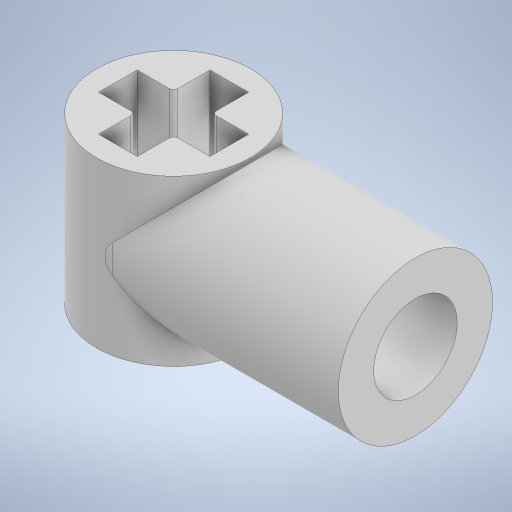
# Autodesk Inventor part: Part2
Saved by Autodesk Inventor 2024 (Build 280153000, 153)
## iProperties
Created: 2023-10-06
Part Number: Part2
Material: Generic
Document SubType Name: Modeling
Designer: kubad
Density: 1 g/cm^3
Appearance: Default
Author: kubad
## iProperties of the stored document Part2_3DPrint.ipt
Created: 2023-10-06
Part Number: Part2_3DPrint
Material: Generic
Document SubType Name: Modeling
Designer: kubad
Density: 1 g/cm^3
Appearance: Default
Author: kubad
Autodesk Inventor part; units mm, degrees
ref_plane "YZ Plane" through (0, 0, 0) normal (1, 0, 0) x (0, 1, 0)
ref_plane "XZ Plane" through (0, 0, 0) normal (0, 1, 0) x (-1, 0, 0)
ref_plane "XY Plane" through (0, 0, 0) normal (0, 0, 1) x (1, 0, 0)
sketch "Sketch1" plane through (0, 0, 0) normal (0, 1, 0) x (-1, 0, 0)
  point P0 (0, 0)
sketch "Sketch2" plane through (0, 0, 0) normal (0, 1, 0) x (-1, 0, 0)
  circle A0 centre (0, 0) radius 3.6
  dimension "d0" = 7.2
  constraints: 1 centre point, 1 coincident
  measures "d0" diameter of A0
extrude "Extrusion1" add sketch "Sketch2" along normal blind 7.7
sketch "Sketch3" plane through (0, 0, 0) normal (0, -1, 0) x (1, 0, 0)
  circle A0 centre (0, 0) radius 3.6 projected
  line L0 (0, 3.6) -> (3.6, 3.6)
  line L1 (3.6, 3.6) -> (3.6, -3.6)
  line L2 (3.6, -3.6) -> (0, -3.6)
  line L3 (0, -3.6) -> (0, 3.6)
  line L4 (3.6, 3.6) -> (11.4, 3.6)
  line L5 (11.4, 3.6) -> (11.4, -3.6)
  line L6 (11.4, -3.6) -> (3.6, -3.6)
  line L7 (3.6, -3.6) -> (3.6, 3.6)
  line L8 (11.4, 3.6) -> (11.3, 3.6)
  line L9 (11.3, 3.6) -> (11.3, -3.6)
  line L10 (11.3, -3.6) -> (11.4, -3.6)
  line L11 (11.4, -3.6) -> (11.4, 3.6)
  dimension "d3" = 7.8
  dimension "d4" = 0.1
  constraints: 24 end point, 6 parallel, 3 horizontal, 3 perpendicular, 1 point on line, 1 vertical alignment, 1 other
  measures "d3" distance of L5.end L6.end
  measures "d4" distance of L10.end L9.end
extrude "Extrusion2" add sketch "Sketch3" against normal blind 7.8 contours L4 L5 L6 L9
sketch "Sketch4" plane through (11.4, 0, 3.6) normal (1, 0, 0) x (0, 0, -1)
  line L0 (3.6, 0) -> (3.6, 0.3)
  line L1 (3.6, 0.3) -> (3.6, 3.9)
  line L2 (3.6, 3.9) -> (3.6, 7.5)
  circle A0 centre (3.6, 3.9) radius 3.6
  dimension "d7" = 0.3
  dimension "d8" = 3.6
  dimension "d9" = 3.6
  constraints: 6 end point, 3 vertical, 1 coincident, 1 vertical alignment, 2 other
  measures "d7" distance of L0.start L0.end
  measures "d8" distance of L0.end L1.end
  measures "d9" distance of L1.end L2.end
extrude "Extrusion3" add sketch "Sketch4" against normal blind 11
fillet "Fillet1" radius 3 1 edges at (0.4, 3.9, 3.6)
fillet "Fillet2" radius 3 2 edges at (0.4, 3.6997, -3.5944) (0.4, 4.1003, -3.5944)
sketch "Sketch5" plane through (11.4, 0, 3.6) normal (1, 0, 0) x (0, 0, -1)
  line L0 (7.2, 0) -> (7.2, 3.9) projected
  line L1 (0, 7.8) -> (7.2, 7.8)
  line L2 (7.2, 7.8) -> (7.2, 0)
  line L3 (7.2, 0) -> (0, 0)
  line L4 (0, 0) -> (0, 7.8)
  point P0 (3.6, 0)
  constraints: 8 end point, 2 parallel, 1 horizontal, 1 perpendicular
extrude "Extrusion4" cut sketch "Sketch5" against normal blind 0.1
sketch "Sketch6" plane through (0, 7.7, 0) normal (0, 1, 0) x (1, 0, 0)
  circle A0 centre (0, 0) radius 3.6 projected
  line L0 (0, -3.6) -> (0, -2.4)
  line L1 (0, 3.6) -> (0, 2.4)
  line L2 (3.6, 0) -> (2.4, 0)
  line L3 (-3.6, 0) -> (-2.4, 0)
  line L4 (0, 2.4) -> (0.9, 2.4)
  line L5 (0, 2.4) -> (-0.9, 2.4)
  line L6 (0, -2.4) -> (0.9, -2.4)
  line L7 (-0.9, 2.4) -> (0.9, 2.4)
  line L8 (0.9, 2.4) -> (0.9, -2.4)
  line L9 (0.9, -2.4) -> (-0.9, -2.4)
  line L10 (-0.9, -2.4) -> (-0.9, 2.4)
  line L11 (-2.4, 0) -> (-2.4, 0.9)
  line L12 (2.4, 0) -> (2.4, -0.9)
  line L13 (-2.4, 0.9) -> (2.4, 0.9)
  line L14 (2.4, 0.9) -> (2.4, -0.9)
  line L15 (2.4, -0.9) -> (-2.4, -0.9)
  line L16 (-2.4, -0.9) -> (-2.4, 0.9)
  point P0 (-0.9, -0.9)
  point P1 (-0.9, 0.9)
  point P2 (0.9, -0.9)
  point P3 (0.9, 0.9)
  dimension "d16" = 1.2
  dimension "d17" = 1.2
  dimension "d18" = 1.2
  dimension "d19" = 1.2
  dimension "d20" = 0.9
  dimension "d21" = 0.9
  dimension "d22" = 0.9
  dimension "d23" = 0.9
  dimension "d24" = 0.9
  constraints: 34 end point, 7 horizontal, 4 parallel, 4 point on circle, 4 vertical, 2 perpendicular
  measures "d16" distance of L0.start L0.end
  measures "d17" distance of L1.start L1.end
  measures "d18" distance of L2.start L2.end
  measures "d19" distance of L3.start L3.end
  measures "d20" distance of L1.end L4.end
  measures "d21" distance of L1.end L5.end
  measures "d22" distance of L0.end L6.end
  measures "d23" distance of L3.end L11.end
  measures "d24" distance of L2.end L12.end
extrude "Extrusion5" cut sketch "Sketch6" against normal through all contours L11 L13 L10 L15 L16
extrude "Extrusion6" cut sketch "Sketch6" against normal through all contours L12 L15 L8 L13 L14 | L4 L8 L13 L10 L5 | L9 L10 L15 L8 L6 | L15 L10 L13 L8
fillet "Fillet3" radius 0.2 1 edges at (-0.9, 3.85, 0.9)
fillet "Fillet4" radius 0.2 1 edges at (-0.9, 3.85, -0.9)
fillet "Fillet5" radius 0.2 1 edges at (0.9, 3.85, -0.9)
fillet "Fillet6" radius 0.2 1 edges at (0.9, 3.85, 0.9)
sketch "Sketch7" plane through (11.3, 3.9, 0) normal (1, 0, 0) x (0, 0, -1)
  circle A0 centre (0, 0) radius 1
  point P0 (0, -3.9)
  dimension "d33" = 2
  constraints: 1 centre point
  measures "d33" diameter of A0
extrude "Extrusion7" cut sketch "Sketch7" against normal blind 6.5
sketch "Sketch8" plane through (11.3, 3.9, 0) normal (1, 0, 0) x (0, 0, -1)
  line L0 (-2.9498, 0.9535) -> (-1.274, 0.9535) construction
  line L1 (-1.274, 0.9535) -> (-1.274, -1.0465) construction
  line L2 (-1.274, -1.0465) -> (-2.9498, -1.0465) construction
  line L3 (-2.9498, -1.0465) -> (-2.9498, 0.9535) construction
  line L4 (-2.9628, -1.0465) -> (-2.2885, 0.9535)
  line L5 (-2.2885, 0.9535) -> (-1.9612, 0.9535)
  line L6 (-1.9612, 0.9535) -> (-1.2869, -1.0465)
  line L7 (-1.2869, -1.0465) -> (-1.5673, -1.0465)
  line L8 (-1.5673, -1.0465) -> (-1.7488, -0.4874)
  line L9 (-1.7488, -0.4874) -> (-2.5122, -0.4874)
  line L10 (-2.5122, -0.4874) -> (-2.6937, -1.0465)
  line L11 (-2.6937, -1.0465) -> (-2.9628, -1.0465)
  line L12 (-1.8218, -0.2605) -> (-2.1313, 0.6812)
  line L13 (-2.1313, 0.6812) -> (-2.4393, -0.2605)
  line L14 (-2.4393, -0.2605) -> (-1.8218, -0.2605)
  point P0 (0, -3.9)
  constraints: 2 other
extrude "Extrusion8" cut sketch "Sketch8" against normal blind 0.2
sketch "Sketch9" plane through (11.3, 3.9, 0) normal (1, 0, 0) x (0, 0, -1)
  line L0 (-3.0916, -1.2056) -> (-1.159, -1.2056)
  line L1 (-1.159, -1.2056) -> (-1.159, 1.142)
  line L2 (-1.159, 1.142) -> (-3.0916, 1.142)
  line L3 (-3.0916, 1.142) -> (-3.0916, -1.2056)
  point P0 (0, -3.9)
  constraints: 8 end point, 2 parallel, 1 horizontal, 1 perpendicular
extrude "Extrusion9" add sketch "Sketch9" against normal blind 1
sketch "Sketch10" plane through (11.3, 3.9, 0) normal (1, 0, 0) x (0, 0, -1)
  circle A0 centre (0, 0) radius 1.95
  point P0 (0, -3.9)
  dimension "d40" = 3.9
  constraints: 1 centre point
  measures "d40" diameter of A0
extrude "Extrusion10" cut sketch "Sketch10" against normal blind 7
sketch "Sketch11" plane through (0, 7.7, 0) normal (0, 1, 0) x (1, 0, 0)
  line L0 (-2.4, 0.9) -> (-2.4, -0.9) projected
  line L1 (-2.4, -0.9) -> (-2.6, -0.9)
  line L2 (-2.6, -0.9) -> (-2.6, 0.9)
  line L3 (-2.6, 0.9) -> (-2.4, 0.9)
  line L4 (-2.4, 0.9) -> (-2.4, -0.9)
  line L5 (1.1, -0.9) -> (2.4, -0.9) projected
  line L6 (2.4, -0.9) -> (2.6, -0.9)
  line L7 (2.6, -0.9) -> (2.6, 0.9)
  line L8 (2.6, 0.9) -> (2.4, 0.9)
  line L9 (2.4, 0.9) -> (2.4, -0.9)
  line L10 (0.9, 2.4) -> (-0.9, 2.4) projected
  line L11 (-0.9, 2.4) -> (0.9, 2.4)
  line L12 (0.9, 2.4) -> (0.9, 2.6)
  line L13 (0.9, 2.6) -> (-0.9, 2.6)
  line L14 (-0.9, 2.6) -> (-0.9, 2.4)
  line L15 (-0.9, -1.1) -> (-0.9, -2.4) projected
  line L16 (-0.9, -2.4) -> (0.9, -2.4)
  line L17 (0.9, -2.4) -> (0.9, -2.6)
  line L18 (0.9, -2.6) -> (-0.9, -2.6)
  line L19 (-0.9, -2.6) -> (-0.9, -2.4)
  point P0 (0, 0)
  dimension "d43" = 0.2
  dimension "d44" = 0.2
  dimension "d45" = 0.2
  dimension "d46" = 0.2
  constraints: 32 end point, 8 parallel, 4 horizontal, 4 perpendicular
  measures "d43" distance of L2.end L3.end
  measures "d44" distance of L8.end L7.end
  measures "d45" distance of L12.end L11.end
  measures "d46" distance of L16.end L17.end
extrude "Extrusion11" cut sketch "Sketch11" against normal through all contours L0 L1 L2 L3
extrude "Extrusion12" cut sketch "Sketch11" against normal through all contours L10 L14 L13 L12
extrude "Extrusion13" cut sketch "Sketch11" against normal through all contours L16 L17 L18 L19
extrude "Extrusion14" cut sketch "Sketch11" against normal through all contours L9 L8 L7 L6
body "Solid1"
